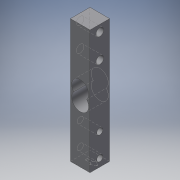
# Autodesk Inventor part: LoadCell
Saved by Autodesk Inventor 2016 (Build 200138000, 138)
## iProperties
Created: 2016-12-23
Part Number: LoadCell
Material: Generic
Document SubType Name: Modeling
Designer: inorn
Density: 1 g/cm^3
Appearance: Default
Author: inorn
Autodesk Inventor part; units mm, degrees
ref_plane "YZ Plane" through (0, 0, 0) normal (1, 0, 0) x (0, 1, 0)
ref_plane "XZ Plane" through (0, 0, 0) normal (0, 1, 0) x (-1, 0, 0)
ref_plane "XY Plane" through (0, 0, 0) normal (0, 0, 1) x (1, 0, 0)
sketch "Sketch1" plane through (0, 0, 0) normal (0, 1, 0) x (-1, 0, 0)
  line L0 (0, 0) -> (12.7, 0)
  line L1 (12.7, 0) -> (12.7, -80)
  line L2 (12.7, -80) -> (0, -80)
  line L3 (0, -80) -> (0, 0)
  circle A0 centre (6.35, -36.5) radius 5.5
  circle A1 centre (6.35, -43.5) radius 5.5
  line L4 (6.35, -36.5) -> (6.35, -43.5) construction
  point P0 (6.35, -40)
  point P1 (0, -40)
  point P2 (6.35, -80)
  dimension "d0" = 12.7
  dimension "d1" = 80
  dimension "d2" = 11
  dimension "d3" = 11
  dimension "d4" = 7
  constraints: 10 end point, 3 midpoint, 2 centre point, 2 parallel, 1 horizontal, 1 horizontal alignment, 1 perpendicular, 1 vertical, 1 vertical alignment
  measures "d0" distance of L1.end L2.end
  measures "d1" distance of L0.end L1.end
  measures "d2" diameter of A0
  measures "d3" diameter of A1
  measures "d4" distance of L4.end L4.start
extrude "Extrusion1" add sketch "Sketch1" along normal blind 12.7
sketch "Sketch2" plane through (-12.7, 0, -80) normal (-1, 0, 0) x (0, 0, 1)
  line L0 (40, 0) -> (40, 12.7) projected
  line L1 (40, 6.35) -> (20, 6.35) construction
  line L2 (20, 6.35) -> (5, 6.35) construction
  circle A0 centre (5, 6.35) radius 2
  circle A1 centre (20, 6.35) radius 2
  line L3 (40, 6.35) -> (60, 6.35) construction
  line L4 (60, 6.35) -> (75, 6.35) construction
  circle A2 centre (60, 6.35) radius 2.5
  circle A3 centre (75.6534, 6.35) radius 2.5
  point P0 (80, 0)
  dimension "d7" = 20
  dimension "d8" = 15
  dimension "d9" = 4
  dimension "d10" = 4
  dimension "d11" = 5
  dimension "d12" = 5
  constraints: 8 end point, 4 centre point, 3 coincident, 2 horizontal, 2 symmetric about line, 1 midpoint
  measures "d7" distance of L1.start L1.end
  measures "d8" distance of L1.end L2.end
  measures "d9" diameter of A0
  measures "d10" diameter of A1
  measures "d11" diameter of A2
  measures "d12" diameter of A3
sketch "Sketch3" plane through (0, 0, -80) normal (0, 0, -1) x (-1, 0, 0)
  line L0 (8.7436, 7.084) -> (3.6466, 7.084)
  line L1 (3.6466, 7.084) -> (3.6466, 5.616)
  line L2 (3.6466, 5.616) -> (8.7436, 5.616)
  line L3 (8.7436, 5.616) -> (8.7436, 7.084)
  line L4 (8.7436, 7.084) -> (3.6466, 5.616) construction
  line L5 (3.6466, 7.084) -> (8.7436, 5.616) construction
  line L6 (1.2106, 6.35) -> (4.8647, 8.4597)
  line L7 (4.8647, 8.4597) -> (4.8647, 4.2403)
  line L8 (4.8647, 4.2403) -> (1.2106, 6.35)
  point P0 (0, 0)
  point P1 (6.1951, 6.35)
  point P2 (3.6466, 6.35)
  constraints: 18 end point, 3 midpoint, 2 parallel, 1 horizontal, 1 perpendicular, 7 other
extrude "Extrusion2" cut sketch "Sketch3" against normal blind 0.1
extrude "Extrusion3" cut sketch "Sketch2" against normal through all
body "Solid1"
